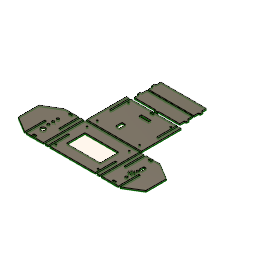
monochronCase v1 (Autodesk Fusion 360 design; units mm, degrees)
Autodesk Fusion 360 part; units mm, degrees
sketch "Sketch1" plane through (0, 0, 0) normal (0, 1, 0) x (1, 0, 0)
  line L0 (77.2897, -234.7425) -> (83.6397, -234.7425)
  line L1 (83.6397, -234.7425) -> (83.6397, -193.0626)
  line L2 (83.6397, -193.0626) -> (86.8147, -193.0626)
  line L3 (86.8147, -193.0626) -> (86.8147, -234.7882)
  line L4 (86.8147, -234.7882) -> (182.0647, -234.7882)
  line L5 (182.0647, -234.7882) -> (182.0647, -193.0626)
  line L6 (182.0647, -193.0626) -> (185.2397, -193.0626)
  line L7 (185.2397, -193.0626) -> (185.2397, -234.7422)
  line L8 (185.2397, -234.7422) -> (191.5897, -234.7422)
  line L9 (191.5897, -234.7422) -> (191.5897, -151.3611)
  line L10 (191.5897, -151.3611) -> (77.2897, -151.3611)
  line L11 (77.2897, -151.3611) -> (77.2897, -234.7425)
  line L12 (99.4522, -173.8094) -> (169.4523, -173.8094)
  line L13 (169.4523, -173.8094) -> (169.4523, -211.8093)
  line L14 (169.4523, -211.8093) -> (99.4522, -211.8093)
  line L15 (99.4522, -211.8093) -> (99.4522, -173.8094)
  circle A0 centre (90.4502, -160.3187) radius 1.5875
  circle A1 centre (178.45, -160.3187) radius 1.5875
  circle A2 centre (178.45, -225.3188) radius 1.5875
  circle A3 centre (90.4486, -225.3188) radius 1.5875
  spline S0 degree 3 poles (43.7599, -196.657) (43.7603, -195.2542) (44.8978, -194.1176) (46.3001, -194.1176) knots 0 0 0 0 1 1 1 1
  spline S1 degree 3 poles (46.3001, -194.1176) (47.7027, -194.1176) (48.8399, -195.2542) (48.8399, -196.657) knots 0 0 0 0 1 1 1 1
  spline S2 degree 3 poles (48.8399, -196.657) (48.8399, -198.0602) (47.7027, -199.1972) (46.3003, -199.1972) knots 0 0 0 0 1 1 1 1
  spline S3 degree 3 poles (46.3003, -199.1972) (44.8975, -199.1972) (43.7599, -198.0602) (43.7599, -196.657) knots 0 0 0 0 1 1 1 1
  spline S4 degree 3 poles (43.7599, -186.7154) (43.7603, -185.313) (44.8978, -184.1763) (46.3001, -184.1763) knots 0 0 0 0 1 1 1 1
  spline S5 degree 3 poles (46.3001, -184.1763) (47.7027, -184.1763) (48.8399, -185.313) (48.8399, -186.7154) knots 0 0 0 0 1 1 1 1
  spline S6 degree 3 poles (48.8399, -186.7154) (48.8399, -188.1184) (47.7027, -189.2553) (46.3003, -189.2553) knots 0 0 0 0 1 1 1 1
  spline S7 degree 3 poles (46.3003, -189.2553) (44.8975, -189.2553) (43.7599, -188.1184) (43.7599, -186.7154) knots 0 0 0 0 1 1 1 1
  spline S8 degree 3 poles (43.7599, -176.8185) (43.7603, -175.4158) (44.8975, -174.2791) (46.3001, -174.2791) knots 0 0 0 0 1 1 1 1
  spline S9 degree 3 poles (46.3001, -174.2791) (47.7021, -174.2791) (48.8399, -175.4158) (48.8399, -176.8185) knots 0 0 0 0 1 1 1 1
  spline S10 degree 3 poles (48.8399, -176.8185) (48.8393, -178.2218) (47.7027, -179.3585) (46.3003, -179.3585) knots 0 0 0 0 1 1 1 1
  spline S11 degree 3 poles (46.3003, -179.3585) (44.8975, -179.3585) (43.7599, -178.2213) (43.7599, -176.8185) knots 0 0 0 0 1 1 1 1
  line L16 (74.2394, -234.8029) -> (74.2394, -151.4043)
  line L17 (74.2394, -151.4043) -> (67.8889, -151.416)
  line L18 (67.8889, -151.416) -> (67.8891, -193.1767)
  line L19 (67.8891, -193.1767) -> (64.7144, -193.1767)
  line L20 (64.7144, -193.1767) -> (64.7144, -151.3792)
  line L21 (64.7144, -151.3792) -> (46.5884, -151.3789)
  line L22 (46.5884, -151.3789) -> (35.0843, -151.3477)
  line L23 (35.0843, -151.3477) -> (1.452, -171.6552)
  line L24 (1.452, -171.6552) -> (1.452, -214.5266)
  line L25 (1.452, -214.5266) -> (35.1277, -234.888)
  line L26 (35.1277, -234.888) -> (35.0667, -192.9247)
  line L27 (35.0667, -192.9247) -> (38.2412, -192.9254)
  line L28 (38.2412, -192.9254) -> (38.272, -234.9655)
  line L29 (38.272, -234.9655) -> (74.2394, -234.8029)
  line L30 (194.4919, -234.8029) -> (194.4919, -151.4043)
  line L31 (194.4919, -151.4043) -> (200.8426, -151.416)
  line L32 (200.8426, -151.416) -> (200.8421, -193.2036)
  line L33 (200.8421, -193.2036) -> (204.0169, -193.2036)
  line L34 (204.0169, -193.2036) -> (204.0169, -151.3792)
  line L35 (204.0169, -151.3792) -> (222.1431, -151.3789)
  line L36 (222.1431, -151.3789) -> (233.6472, -151.3477)
  line L37 (233.6472, -151.3477) -> (267.2791, -171.6552)
  line L38 (267.2791, -171.6552) -> (267.2791, -214.5266)
  line L39 (267.2791, -214.5266) -> (233.6038, -234.888)
  line L40 (233.6038, -234.888) -> (233.6648, -192.8388)
  line L41 (233.6648, -192.8388) -> (230.49, -192.8396)
  line L42 (230.49, -192.8396) -> (230.4593, -234.9655)
  line L43 (230.4593, -234.9655) -> (194.4919, -234.8029)
  circle A4 centre (222.7212, -210.5995) radius 2.667
  circle A5 centre (220.4415, -191.0415) radius 0.508
  circle A6 centre (220.4415, -203.7415) radius 0.508
  circle A7 centre (226.7915, -197.3915) radius 0.508
  circle A8 centre (214.0915, -197.3915) radius 0.508
  ellipse E0 centre (224.9317, -192.9013) end of major axis (224.5725, -192.5421) minor radius 0.5081
  ellipse E1 centre (215.9513, -201.8817) end of major axis (215.5921, -201.5225) minor radius 0.5081
  ellipse E2 centre (224.9317, -201.8817) end of major axis (224.5725, -201.5225) minor radius 0.5081
  ellipse E3 centre (215.9513, -192.9013) end of major axis (215.5921, -192.5421) minor radius 0.5081
  ellipse E4 centre (222.2437, -193.041) end of major axis (221.7744, -192.8466) minor radius 0.5079
  ellipse E5 centre (216.1934, -195.6318) end of major axis (215.7242, -195.4375) minor radius 0.5079
  ellipse E6 centre (218.6394, -201.742) end of major axis (218.1701, -201.5477) minor radius 0.5079
  ellipse E7 centre (224.6897, -199.1512) end of major axis (224.2205, -198.9569) minor radius 0.5079
  ellipse E8 centre (218.6394, -193.041) end of major axis (218.1701, -193.2354) minor radius 0.5079
  ellipse E9 centre (216.1934, -199.1512) end of major axis (215.7241, -199.3456) minor radius 0.5079
  ellipse E10 centre (222.2437, -201.742) end of major axis (221.7744, -201.9364) minor radius 0.5079
  ellipse E11 centre (224.6897, -195.6318) end of major axis (224.2204, -195.8262) minor radius 0.5079
  circle A9 centre (220.4415, -194.4705) radius 0.508
  circle A10 centre (217.5205, -197.3915) radius 0.508
  circle A11 centre (220.4415, -200.3125) radius 0.508
  circle A12 centre (223.3625, -197.3915) radius 0.508
  ellipse E12 centre (222.507, -195.326) end of major axis (222.1478, -194.9667) minor radius 0.5081
  ellipse E13 centre (218.376, -195.326) end of major axis (218.0167, -194.9667) minor radius 0.5081
  ellipse E14 centre (218.376, -199.4571) end of major axis (218.0167, -199.0978) minor radius 0.5081
  ellipse E15 centre (222.507, -199.4571) end of major axis (222.1478, -199.0978) minor radius 0.5081
  ellipse E16 centre (220.422, -197.3351) end of major axis (219.9528, -197.1408) minor radius 0.5079
  line L44 (86.8563, -32.2687) -> (182.0715, -32.2687)
  line L45 (182.0715, -32.2687) -> (182.0715, -42.3781)
  line L46 (182.0715, -42.3781) -> (185.2361, -42.3819)
  line L47 (185.2361, -42.3819) -> (185.229, -48.7695)
  line L48 (185.229, -48.7695) -> (182.0835, -48.7782)
  line L49 (182.0835, -48.7782) -> (182.0715, -58.9275)
  line L50 (182.0715, -58.9275) -> (137.5827, -58.9298)
  line L51 (137.5827, -58.9298) -> (137.5761, -60.6895)
  line L52 (137.5761, -60.6895) -> (131.3134, -60.6903)
  line L53 (131.3134, -60.6903) -> (131.3152, -58.9557)
  line L54 (131.3152, -58.9557) -> (86.8563, -58.8602)
  line L55 (86.8563, -58.8602) -> (86.8563, -48.6976)
  line L56 (86.8563, -48.6976) -> (83.7677, -48.6976)
  line L57 (83.7677, -48.6976) -> (83.7372, -42.3581)
  line L58 (83.7372, -42.3581) -> (86.8563, -42.3794)
  line L59 (86.8563, -42.3794) -> (86.8563, -32.2687)
  line L60 (191.5897, -65.0471) -> (185.2397, -65.0471)
  line L61 (185.2397, -65.0471) -> (185.2397, -106.7267)
  line L62 (185.2397, -106.7267) -> (182.0647, -106.7267)
  line L63 (182.0647, -106.7267) -> (182.0647, -65.0011)
  line L64 (182.0647, -65.0011) -> (86.8147, -65.0011)
  line L65 (86.8147, -65.0011) -> (86.8147, -106.7267)
  line L66 (86.8147, -106.7267) -> (83.6397, -106.7267)
  line L67 (83.6397, -106.7267) -> (83.6397, -65.0471)
  line L68 (83.6397, -65.0471) -> (77.2897, -65.0471)
  line L69 (77.2897, -65.0471) -> (77.2897, -148.4282)
  line L70 (77.2897, -148.4282) -> (191.5897, -148.4282)
  line L71 (191.5897, -148.4282) -> (191.5897, -65.0471)
  circle A13 centre (178.4292, -73.9587) radius 1.5875
  circle A14 centre (90.4291, -73.9587) radius 1.5875
  circle A15 centre (90.4291, -138.9588) radius 1.5875
  circle A16 centre (178.4307, -138.9588) radius 1.5875
  line L72 (125.9202, -82.8205) -> (146.1256, -82.8205)
  line L73 (146.1256, -82.8205) -> (146.1256, -87.6832)
  line L74 (146.1256, -87.6832) -> (125.9202, -87.6832)
  line L75 (125.9202, -87.6832) -> (125.9202, -82.8205)
  line L76 (119.5535, -116.8291) -> (127.1735, -116.8291)
  line L77 (127.1735, -116.8291) -> (127.1735, -129.5291)
  line L78 (127.1735, -129.5291) -> (119.5535, -129.5291)
  line L79 (119.5535, -129.5291) -> (119.5535, -116.8291)
  line L80 (131.2647, -67.4891) -> (137.6147, -67.4891)
  line L81 (137.6147, -67.4891) -> (137.6147, -70.5371)
  line L82 (137.6147, -70.5371) -> (131.2647, -70.5371)
  line L83 (131.2647, -70.5371) -> (131.2647, -67.4891)
  line L84 (48.3062, -153.8338) -> (54.6562, -153.8338)
  line L85 (54.6562, -153.8338) -> (54.6562, -156.8818)
  line L86 (54.6562, -156.8818) -> (48.3062, -156.8818)
  line L87 (48.3062, -156.8818) -> (48.3062, -153.8338)
  line L88 (214.092, -153.8338) -> (220.442, -153.8338)
  line L89 (220.442, -153.8338) -> (220.442, -156.8818)
  line L90 (220.442, -156.8818) -> (214.092, -156.8818)
  line L91 (214.092, -156.8818) -> (214.092, -153.8338)
  line L92 (48.3062, -229.0122) -> (54.6562, -229.0122)
  line L93 (54.6562, -229.0122) -> (54.6562, -232.0602)
  line L94 (54.6562, -232.0602) -> (48.3062, -232.0602)
  line L95 (48.3062, -232.0602) -> (48.3062, -229.0122)
  line L96 (214.0786, -229.0122) -> (220.4286, -229.0122)
  line L97 (220.4286, -229.0122) -> (220.4286, -232.0602)
  line L98 (220.4286, -232.0602) -> (214.0786, -232.0602)
  line L99 (214.0786, -232.0602) -> (214.0786, -229.0122)
  line L100 (86.8563, -3.0586) -> (182.0715, -3.0586)
  line L101 (182.0715, -3.0586) -> (182.0715, -13.168)
  line L102 (182.0715, -13.168) -> (185.2361, -13.172)
  line L103 (185.2361, -13.172) -> (185.229, -19.5594)
  line L104 (185.229, -19.5594) -> (182.0835, -19.5682)
  line L105 (182.0835, -19.5682) -> (182.0715, -29.7175)
  line L106 (182.0715, -29.7175) -> (86.8563, -29.6502)
  line L107 (86.8563, -29.6502) -> (86.8563, -19.4876)
  line L108 (86.8563, -19.4876) -> (83.7677, -19.4876)
  line L109 (83.7677, -19.4876) -> (83.7372, -13.1481)
  line L110 (83.7372, -13.1481) -> (86.8563, -13.1695)
  line L111 (86.8563, -13.1695) -> (86.8563, -3.0586)
  line L112 (51.2422, -187.5165) -> (51.6098, -187.4587)
  spline S12 degree 3 poles (51.6253, -187.0629) (51.5202, -187.0128) (51.4398, -186.9429) (51.3855, -186.854) knots 0 0 0 0 1 1 1 1
  spline S13 degree 3 poles (51.3713, -186.2882) (51.4158, -186.2042) (51.4772, -186.1351) (51.5541, -186.08) knots 0 0 0 0 1 1 1 1
  spline S14 degree 3 poles (52.1806, -188.2214) (51.8949, -188.2214) (51.6776, -188.1621) (51.528, -188.0436) knots 0 0 0 0 1 1 1 1
  spline S15 degree 3 poles (51.528, -188.0436) (51.3784, -187.9251) (51.2831, -187.7494) (51.2422, -187.5165) knots 0 0 0 0 1 1 1 1
  line L113 (222.9213, -173.9008) -> (226.7819, -173.9008)
  arc A17 (226.7819, -173.9008) -> (227.6092, -174.7281) centre (226.7819, -174.7281) cw
  line L114 (227.6092, -174.7281) -> (227.6092, -183.0736)
  arc A18 (227.6092, -183.0736) -> (226.7819, -183.9009) centre (226.7819, -183.0736) cw
  line L115 (226.7819, -183.9009) -> (222.9213, -183.9009)
  arc A19 (222.9213, -183.9009) -> (222.094, -183.0736) centre (222.9213, -183.0736) cw
  line L116 (222.094, -183.0736) -> (222.094, -174.7281)
  arc A20 (222.094, -174.7281) -> (222.9213, -173.9008) centre (222.9213, -174.7281) cw
  circle A21 centre (223.966, -188.1899) radius 2.54
  circle A22 centre (48.8485, -210.3023) radius 4.7624
extrude "Extrude1" add sketch "Sketch1" along normal blind 3 contours L0 L1 L2 L3 L4 L5 L6 L7 L8 L9 L10 L11 makes body 1
extrude "Extrude2" add sketch "Sketch1" along normal blind 3 separate body contours L30 L31 L32 L33 L34 L35 L36 L37 L38 L39 L40 L41 L42 L43 makes body 2
extrude "Extrude3" add sketch "Sketch1" along normal blind 3 separate body contours L16 L17 L18 L19 L20 L21 L22 L23 L24 L25 L26 L27 L28 L29 makes body 3
extrude "Extrude4" add sketch "Sketch1" along normal blind 3 separate body contours L60 L61 L62 L63 L64 L65 L66 L67 L68 L69 L70 L71 makes body 4
extrude "Extrude5" add sketch "Sketch1" along normal blind 3 separate body contours L44 L45 L46 L47 L48 L49 L50 L51 L52 L53 L54 L55 L56 L57 L58 L59 makes body 5
extrude "Extrude6" add sketch "Sketch1" along normal blind 3 separate body contours L100 L101 L102 L103 L104 L105 L106 L107 L108 L109 L110 L111 makes body 6
equation "paksuus = 3 mm"
equation "d4 = paksuus"
equation "d6 = paksuus"
equation "d8 = paksuus"
equation "d10 = paksuus"
equation "d12 = paksuus"
named bodies: "etuseina", "vasen", "oikeia", "takaseina", "yla", "ala"
